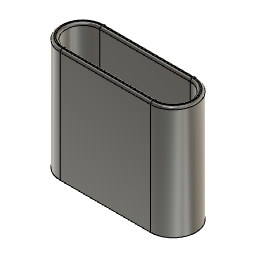
Pencil Holder v1 (Autodesk Fusion 360 design; units mm, degrees)
Autodesk Fusion 360 part; units mm, degrees
sketch "Sketch1" plane through (0, 0, 0) normal (0, 0, 1) x (1, 0, 0)
  line L0 (-50, 0) -> (-50, 30)
  line L1 (-50, 30) -> (50, 30)
  line L2 (50, 30) -> (50, 0)
  line L3 (50, 0) -> (-50, 0)
  constraint perpendicular L0 L1
  constraint parallel L0 L2
  constraint parallel L1 L3
  constraint vertical L0
extrude "Extrude1" add sketch "Sketch1" along normal blind 10 makes body 1
revolve "Revolve1" add 1 faces at (-16.6667, 10, 10) angle 180 about axis through (50, 30, 10) along (-1, 0, 0) on bodies 1 bodies 1
extrude "Extrude2" cut 1 faces at (16.6667, 0, 3.3333) along direction (0, 1, 0) blind 30 on bodies 1 bodies 1
thread "Thread1" "ISO Metric profile 80.0 M80x6 6g" major diameter 79.62 minor diameter 72.736 pitch 6 angle 60 resizes the face on face at (-16.6667, 49.8506, 32.4934) on bodies 1
thread "Thread2" "ISO Metric profile 40.0 M40x3 6g" major diameter 39.7645 minor diameter 36.3299 pitch 3 angle 60 resizes the face on face at (16.6667, 69.7605, 11.9844) on bodies 1
sketch "Sketch1 (2)" plane through (0, 0, 0) normal (0, 0, 1) x (1, 0, 0) in component "Pencil Holder"
  line L0 (-25, -10) -> (25, -10)
  line L1 (25, -10) -> (25, 10)
  line L2 (25, 10) -> (-25, 10)
  line L3 (-25, 10) -> (-25, -10)
  circle A0 centre (-25, 0) radius 10
  circle A1 centre (25, 0) radius 10
  dimension "d9" = 20
  constraint horizontal L0
  constraint vertical L1
  constraint horizontal L2
  constraint vertical L3
  constraint coincident L2.end A0
  constraint tangent L2 A0
  constraint coincident L0.start A0
  constraint coincident L0.end A1
  constraint tangent L0 A1
  constraint coincident L1.end A1
  measures "d9" diameter of A1
extrude "Extrude1'" add sketch "Sketch1 (2)" along normal blind 50 separate body makes body 2 in component "Pencil Holder"
shell "Shell1" thickness 1 removed faces 1 at (8.3333, -3.3333, 50) on bodies 2 in component "Pencil Holder"
sketch "Sketch1 (3)" plane through (0, 0, 0) normal (0, 0, 1) x (1, 0, 0) in component "Pencil Holder 2"
sketch "Sketch2" plane through (0, 0, 0) normal (0, 0, 1) x (1, 0, 0) in component "Pencil Holder 2"
  line L0 (40.0899, 30) -> (-39.9101, 30)
  line L1 (-39.9101, 30) -> (-39.9101, -10)
  line L2 (-39.9101, -10) -> (40.0899, -10)
  line L3 (40.0899, -10) -> (40.0899, 30)
  circle A0 centre (40.0899, 10) radius 20
  circle A1 centre (-39.9101, 10) radius 20
  dimension "d10" = 80
  dimension "d11" = 80
  constraint horizontal L0
  constraint vertical L1
  constraint horizontal L2
  constraint vertical L3
  constraint coincident L0.start A0
  constraint tangent L0 A0
  constraint coincident L2.end A0
  constraint coincident L0.end A1
  constraint tangent L0 A1
  constraint coincident L1.end A1
  measures "d10" distance of L0.start L0.end
  measures "d11" distance of L2.end L0
extrude "Extrude1''" add sketch "Sketch2" along normal blind 100 separate body makes body 3 in component "Pencil Holder 2"
shell "Shell1'" thickness 5 removed faces 1 at (13.4232, 3.3333, 100) on bodies 3 in component "Pencil Holder 2"
fillet "Fillet1" radius 2 4 edges at (-59.9101, 10, 100) (0.0899, -10, 100) (60.0899, 10, 100) (0.0899, 30, 100) on bodies 3 in component "Pencil Holder 2"
fillet "Fillet2" radius 2 4 edges at (0.0899, 25, 100) (55.0899, 10, 100) (0.0899, -5, 100) (-54.9101, 10, 100) on bodies 3 in component "Pencil Holder 2"
component "Pencil Holder" placed x (1, 0, 0) y (0, 1, 0) z (0, 0, 1) at (2.5883, 1.2459, 2.9225)
component "Pencil Holder 2" placed x (1, 0, 0) y (0, 1, 0) z (0, 0, 1) at (0, 0, 0)
